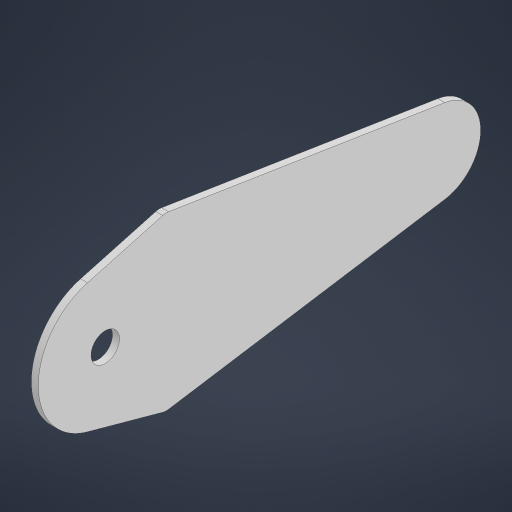
# Autodesk Inventor part: plate
Saved by Autodesk Inventor 2023 (Build 270158000, 158)
## iProperties
Created: 2023-02-24
Part Number: plate
Material: Generic
Document SubType Name: Modeling
Designer: ralph
Density: 1 g/cm^3
Appearance: Default
Author: ralph
Autodesk Inventor part; units mm, degrees
ref_plane "YZ Plane" through (0, 0, 0) normal (1, 0, 0) x (0, 1, 0)
ref_plane "XZ Plane" through (0, 0, 0) normal (0, 1, 0) x (-1, 0, 0)
ref_plane "XY Plane" through (0, 0, 0) normal (0, 0, 1) x (1, 0, 0)
sketch "Sketch1" plane through (0, 0, 0) normal (1, 0, 0) x (0, 1, 0)
  line L0 (-85.3041, -13.4634) -> (-38.3671, -310.8554)
  circle A0 centre (-65.7313, -56.0129) radius 12.7
  line L1 (-59.036, 16.234) -> (-77.9768, -52.6455)
  line L2 (59.036, 16.234) -> (77.9768, -52.6455)
  circle A1 centre (65.7313, -56.0129) radius 12.7
  line L3 (85.3041, -13.4634) -> (38.3671, -310.8554)
  circle A2 centre (0, -304.8) radius 38.842
  circle A3 centre (0, 0) radius 61.2274
  circle A4 centre (0, 0) radius 13.0175
  circle A5 centre (0, -304.8) radius 13.0175
  point P0 (0, 0)
  point P1 (-78.2761, -57.9928)
  point P2 (-38.3671, -310.8554)
  point P3 (38.3671, -310.8554)
  point P4 (78.2761, -57.9928)
  dimension "d0" = 25.4
  dimension "d1" = 26.035
  dimension "d2" = 26.035
  constraints: 8 end point, 6 centre point, 2 coincident
  measures "d0" diameter of A1
  measures "d1" diameter of A4
  measures "d2" diameter of A5
extrude "Extrusion1" add sketch "Sketch1" along normal blind 6.35 contours A0 L1 A3 L2 A1 L3 A2 L0 | A0 | A2 | A3 | A1 | A5
body "Solid1"
